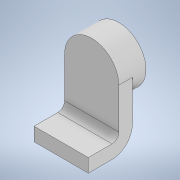
# Autodesk Inventor part: SupportFixture
Saved by Autodesk Inventor 2022.2 (Build 262287030, 287C)
## iProperties
Created: 2023-04-03
Part Number: SupportFixture
Material: Generic
Document SubType Name: Modeling
Designer: jak27277
Density: 1 g/cm^3
Appearance: Default
Author: jak27277
Autodesk Inventor part; units mm, degrees
ref_plane "YZ Plane" through (0, 0, 0) normal (1, 0, 0) x (0, 1, 0)
ref_plane "XZ Plane" through (0, 0, 0) normal (0, 1, 0) x (-1, 0, 0)
ref_plane "XY Plane" through (0, 0, 0) normal (0, 0, 1) x (1, 0, 0)
sketch "Sketch1" plane through (0, 0, 0) normal (0, 0, 1) x (1, 0, 0)
  circle A0 centre (0, 0) radius 50.8
  dimension "d0" = 101.6
  constraints: 1 centre point, 1 coincident
  measures "d0" diameter of A0
extrude "Extrusion1" add sketch "Sketch1" along normal blind 50.8
sketch "Sketch2" plane through (0, 0, 0) normal (1, 0, 0) x (0, 1, 0)
  line L0 (50.8, 50.8) -> (-50.8, 50.8) projected
  line L1 (0, 50.8) -> (-76.2, 50.8)
  arc A0 (-88.9, 63.5) -> (-76.2, 50.8) centre (-76.2, 63.5) ccw
  line L2 (-88.9, 63.5) -> (-88.9, 107.95)
  line L3 (0, 25.4) -> (-76.2, 25.4)
  arc A1 (-114.3, 63.5) -> (-76.2, 25.4) centre (-76.2, 63.5) ccw
  line L4 (-114.3, 63.5) -> (-114.3, 107.95)
  line L5 (-88.9, 107.95) -> (-114.3, 107.95)
  line L6 (-114.3, 107.95) -> (-127, 107.95) construction
  line L7 (0, 50.8) -> (0, 25.4)
  point P0 (0, 0)
  dimension "d3" = 57.15
  dimension "d4" = 12.7
  dimension "d5" = 25.4
  dimension "d6" = 38.1
  dimension "d7" = 127
  constraints: 14 end point, 4 point on circle, 3 horizontal, 2 centre point, 2 tangent, 1 midpoint, 1 perpendicular, 1 vertical, 2 other
  measures "d3" distance from line of L2.end L1
  measures "d4" radius of A0
  measures "d5" distance between parallel lines of L3 L1
  measures "d6" distance from line of L6.end L2
  measures "d7" horizontal distance of L6.end point (0, 0)
extrude "Extrusion2" add sketch "Sketch2" along normal mid plane 101.6
body "Solid1"
